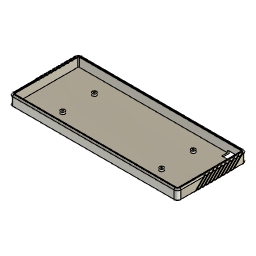
SpeedTray (Autodesk Fusion 360 design; units mm, degrees)
Autodesk Fusion 360 part; units mm, degrees
note: some values were not read from the file. Set by a fixed rule: which sketch regions a step uses.
sketch "Outline Sketch" plane through (0, 0, 0) normal (0, 0, 1) x (1, 0, 0)
  line L0 (16.7505, 7.3816) -> (212.013, 7.3816) construction
  line L1 (212.013, 7.3816) -> (212.013, 83.5816) construction
  line L2 (212.013, 83.5816) -> (16.7505, 83.5816) construction
  line L3 (16.7505, 83.5816) -> (16.7505, 7.3816) construction
  line L4 (212.513, 84.0816) -> (16.2505, 84.0816)
  line L5 (16.2505, 84.0816) -> (16.2505, 6.8816)
  line L6 (16.2505, 6.8816) -> (212.513, 6.8816)
  line L7 (212.513, 6.8816) -> (212.513, 84.0816)
  line L8 (13.0505, 3.6816) -> (215.713, 3.6816)
  line L9 (215.713, 3.6816) -> (215.713, 87.2816)
  line L10 (215.713, 87.2816) -> (13.0505, 87.2816)
  line L11 (13.0505, 87.2816) -> (13.0505, 3.6816)
  dimension "d1" = 195.2625
  dimension "d2" = 76.2
  dimension "d3" = 0.5
  dimension "d4" = 3.7
  constraint horizontal L0
  constraint vertical L1
  constraint horizontal L2
  constraint vertical L3
  measures "d1" distance of L0.start L0.end
  measures "d2" distance of L0.start L2.end
extrude "Extrude1" add sketch "Outline Sketch" along normal blind 8.6
sketch "Angle Sketch" plane through (215.713, 0, 0) normal (1, 0, 0) x (0, 1, 0)
  line L0 (3.6816, 0) -> (87.2816, 0)
  line L1 (87.2816, 0) -> (87.2816, 8.6)
  line L2 (87.2816, 8.6) -> (3.6816, 8.6)
  line L3 (3.6816, 8.6) -> (3.6816, 0)
  line L4 (3.6816, -4.2) -> (87.2816, -4.2)
  dimension "d20" = 4.2
ref_plane "WorkPlane1" through (215.713, 45.4816, -4.2) normal (0, 0, -1) x (0, 1, 0)
sketch "Sketch for Base" plane through (0, 0, 0) normal (0, 0, -1) x (1, 0, 0)
  line L0 (212.513, -6.8816) -> (212.513, -84.0816)
  line L1 (212.513, -84.0816) -> (16.2505, -84.0816)
  line L2 (16.2505, -84.0816) -> (16.2505, -6.8816)
  line L3 (16.2505, -6.8816) -> (212.513, -6.8816)
  line L4 (13.0505, -3.6816) -> (13.0505, -87.2816)
  line L5 (13.0505, -87.2816) -> (215.713, -87.2816)
  line L6 (215.713, -87.2816) -> (215.713, -3.6816)
  line L7 (215.713, -3.6816) -> (13.0505, -3.6816)
  line L8 (13.0505, -87.2816) -> (215.713, -87.2816)
  line L9 (215.713, -87.2816) -> (215.713, -3.6816)
  line L10 (215.713, -3.6816) -> (13.0505, -3.6816)
  line L11 (13.0505, -3.6816) -> (13.0505, -87.2816)
  constraint horizontal L8
  constraint vertical L9
  constraint horizontal L10
  constraint vertical L11
  constraint coincident L6.end L7.start
  constraint coincident L4.end L5.start
extrude "Extrude2" add sketch "Sketch for Base" along normal up to surface (4.2 mm away) contours L0 L1 L2 L3 | L4 L5 L6 L7 L8 L9 L10 L11
sketch "Hole and USB C Cutout Sketch" plane through (0, 0, 0) normal (0, 0, 1) x (-1, 0, 0)
  line L0 (-212.513, -84.0816) -> (-16.2505, -84.0816)
  line L1 (-16.2505, -84.0816) -> (-16.2505, -6.8816)
  line L2 (-16.2505, -6.8816) -> (-212.513, -6.8816)
  line L3 (-212.513, -6.8816) -> (-212.513, -84.0816)
  line L4 (-16.2505, -84.0816) -> (-54.8505, -84.0816) construction
  line L5 (-54.8505, -84.0816) -> (-54.8505, -64.5316) construction
  circle A0 centre (-54.8505, -64.5316) radius 2.5
  line L6 (-212.513, -84.0816) -> (-200.1067, -84.0816)
  line L7 (-195.3817, -87.2816) -> (-204.8317, -87.2816)
  line L8 (-204.8317, -87.2816) -> (-204.8317, -77.4816)
  line L9 (-204.8317, -77.4816) -> (-195.3817, -77.4816)
  line L10 (-195.3817, -77.4816) -> (-195.3817, -87.2816)
  line L11 (-200.1067, -84.0816) -> (-200.1067, -83.5816)
  circle A1 centre (-173.913, -64.5316) radius 2.5
  line L12 (-212.513, -6.8816) -> (-212.513, -84.0816)
  line L13 (-212.513, -84.0816) -> (-16.2505, -84.0816)
  circle A2 centre (-173.913, -26.4316) radius 2.5
  circle A3 centre (-54.8505, -26.4316) radius 2.5
  line L14 (-16.2505, -84.0816) -> (-16.2505, -6.8816)
  line L15 (-16.7505, -7.3816) -> (-212.013, -7.3816)
  line L16 (-16.2505, -6.8816) -> (-212.513, -6.8816)
  dimension "d17" = 38.6
  dimension "d18" = 19.55
  dimension "d19" = 5
  dimension "d21" = 12.4063
  dimension "d22" = 9.45
  dimension "d23" = 4.725
  dimension "d24" = 0.5
  dimension "d25" = 3.7
  dimension "d26" = 9.8
  dimension "d38" = 5
  dimension "d39" = 38.6
  dimension "d40" = 19.55
  dimension "d41" = 5
  dimension "d42" = 5
  dimension "d43" = 38.6
  dimension "d45" = 38.6
  dimension "d46" = 19.55
  dimension "d47" = 19.55
  constraint coincident L0.end L1.start
  constraint perpendicular L1 L4
  constraint perpendicular L4 L5
  constraint coincident L5.end A0.centre
  constraint coincident L0.start L3.end
  constraint perpendicular L3 L6
  constraint horizontal L7
  constraint vertical L8
  constraint horizontal L9
  constraint vertical L10
  constraint perpendicular L6 L11
  measures "d17" distance of L0.end L4.end
  measures "d18" distance of L4.end L5.end
  measures "d19" diameter of A0
  measures "d21" distance of L0.start L6.end
  measures "d22" distance of L8 L10
  measures "d23" distance of L6.end L8
  measures "d24" distance of L6.end L11.end
  measures "d25" distance of L7 L11.end
  measures "d26" distance of L7 L9
  measures "d38" diameter of A1
  measures "d39" distance of A1.centre L12
  measures "d40" distance of A1.centre L13
  measures "d41" diameter of A2
  measures "d42" diameter of A3
  measures "d43" distance of A3.centre L14
  measures "d45" distance of L12 A2.centre
  measures "d46" distance of A2.centre L16
  measures "d47" distance of A3.centre L16
extrude "Extrude3" cut sketch "Hole and USB C Cutout Sketch" along normal blind -6 and the other way blind -0.5 contours L0 L6 L8 L9 L10 L13 | L0 L6 L7 L8 L10 L13
extrude "Extrude4" cut sketch "Hole and USB C Cutout Sketch" against normal blind 2.4 contours L0 L1 L2 L3 L6 L8 L9 L10 L12 L13 L14 L16
fillet "Fillet6" radius 1 4 edges at (16.2505, 6.8816, 3.1) (16.2505, 84.0816, 3.1) (212.513, 84.0816, 3.1) (212.513, 6.8816, 3.1)
hole "Hole1" at (54.8505, 64.5316, 0) direction (0, 0, -1) diameter 1.8 depth 3 tip angle 180
hole "Hole2" at (54.8505, 26.4316, 0) direction (0, 0, -1) diameter 1.8 depth 3 tip angle 180
hole "Hole3" at (173.913, 64.5316, 0) direction (0, 0, -1) diameter 1.8 depth 3 tip angle 180
hole "Hole4" at (173.913, 26.4316, 0) direction (0, 0, -1) diameter 1.8 depth 3 tip angle 180
fillet "Fillet8" radius 4.2 4 edges at (13.0505, 3.6816, 2.2) (13.0505, 87.2816, 2.2) (215.713, 87.2816, 2.2) (215.713, 3.6816, 2.2)
sketch "Decoration Lines" plane through (215.713, 0, 0) normal (1, 0, 0) x (0, 1, 0)
  line L0 (7.8816, 8.6) -> (7.8816, -4.2)
  line L1 (7.8816, -4.2) -> (83.0816, -4.2)
  line L2 (83.0816, -4.2) -> (83.0816, 8.6)
  line L3 (83.0816, 8.6) -> (7.8816, 8.6)
  line L4 (83.0816, 8.6) -> (70.2816, -4.2)
  line L5 (83.0816, 8.6) -> (101.1835, 8.6) construction
  line L6 (83.0816, 8.6) -> (82.3745, 9.3071)
  line L7 (82.3745, 9.3071) -> (68.8674, -4.2)
  line L8 (82.3745, 9.3071) -> (101.4764, 9.3071) construction
  line L9 (68.8674, -4.2) -> (70.2816, -4.2)
  line L10 (78.0816, 8.6) -> (77.3745, 9.3071)
  line L11 (78.0816, 8.6) -> (65.2816, -4.2)
  line L12 (63.8674, -4.2) -> (65.2816, -4.2)
  line L13 (77.3745, 9.3071) -> (63.8674, -4.2)
  line L14 (73.0816, 8.6) -> (72.3745, 9.3071)
  line L15 (73.0816, 8.6) -> (60.2816, -4.2)
  line L16 (58.8674, -4.2) -> (60.2816, -4.2)
  line L17 (72.3745, 9.3071) -> (58.8674, -4.2)
  line L18 (68.0816, 8.6) -> (67.3745, 9.3071)
  line L19 (68.0816, 8.6) -> (55.2816, -4.2)
  line L20 (53.8674, -4.2) -> (55.2816, -4.2)
  line L21 (67.3745, 9.3071) -> (53.8674, -4.2)
  line L22 (63.0816, 8.6) -> (62.3745, 9.3071)
  line L23 (63.0816, 8.6) -> (50.2816, -4.2)
  line L24 (48.8674, -4.2) -> (50.2816, -4.2)
  line L25 (62.3745, 9.3071) -> (48.8674, -4.2)
  line L26 (58.0816, 8.6) -> (57.3745, 9.3071)
  line L27 (58.0816, 8.6) -> (45.2816, -4.2)
  line L28 (43.8674, -4.2) -> (45.2816, -4.2)
  line L29 (57.3745, 9.3071) -> (43.8674, -4.2)
  line L30 (53.0816, 8.6) -> (52.3745, 9.3071)
  line L31 (53.0816, 8.6) -> (40.2816, -4.2)
  line L32 (38.8674, -4.2) -> (40.2816, -4.2)
  line L33 (52.3745, 9.3071) -> (38.8674, -4.2)
  line L34 (48.0816, 8.6) -> (47.3745, 9.3071)
  line L35 (48.0816, 8.6) -> (35.2816, -4.2)
  line L36 (33.8674, -4.2) -> (35.2816, -4.2)
  line L37 (47.3745, 9.3071) -> (33.8674, -4.2)
  line L38 (43.0816, 8.6) -> (42.3745, 9.3071)
  line L39 (43.0816, 8.6) -> (30.2816, -4.2)
  line L40 (28.8674, -4.2) -> (30.2816, -4.2)
  line L41 (42.3745, 9.3071) -> (28.8674, -4.2)
  line L42 (38.0816, 8.6) -> (37.3745, 9.3071)
  line L43 (38.0816, 8.6) -> (25.2816, -4.2)
  line L44 (23.8674, -4.2) -> (25.2816, -4.2)
  line L45 (37.3745, 9.3071) -> (23.8674, -4.2)
  line L46 (83.0816, 8.6) -> (81.6674, 8.6)
  line L47 (82.0816, 7.6) -> (35.6674, 7.6)
  dimension "d139" = 135
  dimension "d140" = 1
  dimension "d141" = 135
  dimension "d144" = -5
  dimension "d145" = 0
  dimension "d170" = 1
  constraint horizontal L5
  constraint coincident L2.end L3.start
  constraint coincident L1 L4.end
  constraint perpendicular L4 L6
  constraint horizontal L8
  constraint coincident L1 L7.end
  constraint coincident L7 L46.end
  constraint coincident L3 L46.end
  constraint perpendicular L2 L47
  constraint coincident L45 L47.end
  constraint coincident L4 L47.start
  measures "d139" angle of L4 L5
  measures "d140" distance of L2.end L6.end
  measures "d141" angle of L7 L8
  measures "d170" distance of L46 L47
fillet "Fillet10" radius 1.5 8 edges at (214.4828, 86.0514, 8.6) (215.713, 45.4816, 8.6) (214.4828, 4.9117, 8.6) (114.3817, 3.6816, 8.6) (14.2806, 4.9117, 8.6) (13.0505, 45.4816, 8.6) (14.2806, 86.0514, 8.6) (114.3817, 87.2816, 8.6)
fillet "Fillet15" radius 1.5 9 edges at (106.3161, 87.2816, -4.2) (14.2806, 86.0514, -4.2) (13.0505, 45.4816, -4.2) (14.2806, 4.9117, -4.2) (114.3817, 3.6816, -4.2) (214.4828, 4.9117, -4.2) (215.713, 45.4816, -4.2) (214.4828, 86.0514, -4.2) (208.1723, 87.2816, -4.2)
chamfer "Chamfer5" distance 0.5 angle 45 8 edges at (114.3817, 84.0816, 8.6) (212.2201, 83.7887, 8.6) (212.513, 45.4816, 8.6) (212.2201, 7.1745, 8.6) (114.3817, 6.8816, 8.6) (16.5434, 7.1745, 8.6) (16.2505, 45.4816, 8.6) (16.5434, 83.7887, 8.6)
extrude "Extrude13" cut sketch "Decoration Lines" against normal blind 1 contours L3 L43 L45 L47 | L1 L43 L44 L45 L47 | L3 L39 L41 L47 | L1 L39 L40 L41 L47 | L3 L35 L37 L47 | L1 L35 L36 L37 L47 | L3 L31 L33 L47 | L1 L31 L32 L33 L47 | L3 L27 L29 L47 | L1 L27 L28 L29 L47 | L3 L23 L25 L47 | L1 L23 L24 L25 L47 | L3 L19 L21 L47 | L1 L19 L20 L21 L47 | L3 L15 L17 L47 | L1 L15 L16 L17 L47 | L3 L11 L13 L47 | L1 L11 L12 L13 L47 | L3 L4 L7 L46 L47 | L1 L4 L7 L9 L47
extrude "Extrude17" cut sketch "Decoration Lines" against normal blind 5 contours L3 L43 L45 L47 | L3 L39 L41 L47 | L3 L35 L37 L47 | L3 L31 L33 L47 | L3 L27 L29 L47 | L3 L23 L25 L47 | L3 L19 L21 L47 | L3 L15 L17 L47 | L3 L11 L13 L47 | L3 L4 L7 L46 L47
extrude "Extrude14" cut sketch "Decoration Lines" along normal blind 1 from surface at -202.6625 contours L3 L43 L45 L47 | L1 L43 L44 L45 L47 | L3 L39 L41 L47 | L1 L39 L40 L41 L47 | L3 L35 L37 L47 | L1 L35 L36 L37 L47 | L3 L31 L33 L47 | L1 L31 L32 L33 L47 | L3 L27 L29 L47 | L1 L27 L28 L29 L47 | L3 L23 L25 L47 | L1 L23 L24 L25 L47 | L3 L19 L21 L47 | L1 L19 L20 L21 L47 | L3 L15 L17 L47 | L1 L15 L16 L17 L47 | L3 L11 L13 L47 | L1 L11 L12 L13 L47 | L3 L4 L7 L46 L47 | L1 L4 L7 L9 L47
extrude "Extrude18" cut sketch "Decoration Lines" along normal blind 5 from surface at -202.6625 contours L3 L43 L45 L47 | L3 L39 L41 L47 | L3 L35 L37 L47 | L3 L31 L33 L47 | L3 L27 L29 L47 | L3 L23 L25 L47 | L3 L19 L21 L47 | L3 L15 L17 L47 | L3 L11 L13 L47 | L3 L4 L7 L46 L47
sketch "Sketch10" plane through (0, 87.2816, 0) normal (0, 1, 0) x (-1, 0, 0)
  line L0 (-211.513, 7.1) -> (-211.513, -2.7)
  line L1 (-204.8317, -2.7) -> (-204.8317, 0.5)
  line L2 (-204.8317, 0.5) -> (-195.3817, 0.5)
  line L3 (-195.3817, 0.5) -> (-195.3817, -2.7)
  line L4 (-17.2505, -2.7) -> (-17.2505, 7.1)
  line L5 (-17.2505, 7.1) -> (-211.513, 7.1)
  line L6 (-211.513, -2.7) -> (-204.8317, -2.7)
  line L7 (-195.3817, -2.7) -> (-17.2505, -2.7)
  line L8 (-204.8317, 0.25) -> (-195.3817, 0.25) construction
  line L9 (-195.3817, 0.25) -> (-195.3817, -3.41) construction
  line L10 (-195.3817, -3.41) -> (-204.8317, -3.41) construction
  line L11 (-204.8317, -3.41) -> (-204.8317, 0.25) construction
  line L12 (-204.8317, -3.41) -> (-195.3817, 0.25) construction
  line L13 (-204.8317, 0.25) -> (-195.3817, -3.41) construction
  line L14 (-196.9317, 2.5) -> (-203.2817, 2.5)
  line L15 (-207.0817, -1.3) -> (-207.0817, -1.86)
  line L16 (-203.2817, -5.66) -> (-196.9317, -5.66)
  line L17 (-193.1317, -1.86) -> (-193.1317, -1.3)
  line L18 (-193.1317, 2.5) -> (-207.0817, -5.66) construction
  line L19 (-207.0817, 2.5) -> (-193.1317, -5.66) construction
  arc A0 (-203.2817, 2.5) -> (-207.0817, -1.3) centre (-203.2817, -1.3) ccw
  arc A1 (-193.1317, -1.3) -> (-196.9317, 2.5) centre (-196.9317, -1.3) ccw
  arc A2 (-196.9317, -5.66) -> (-193.1317, -1.86) centre (-196.9317, -1.86) ccw
  arc A3 (-207.0817, -1.86) -> (-203.2817, -5.66) centre (-203.2817, -1.86) ccw
  point P0 (-200.1067, -1.58)
  dimension "d180" = 9.45
  dimension "d181" = 3.66
  dimension "d182" = 0.25
  dimension "d183" = 13.95
  dimension "d184" = 8.16
  dimension "d185" = 3.8
  constraint horizontal L8
  constraint vertical L9
  constraint horizontal L10
  constraint vertical L11
  constraint collinear L3 L9
  constraint horizontal L14
  constraint perpendicular L14 L15
  constraint parallel L14 L16
  constraint parallel L15 L17
  constraint coincident L18 P0
  constraint coincident L19 P0
  constraint midpoint L12 P0
  constraint coincident L19.start L15
  constraint coincident L19.start L14
  constraint tangent L15 A0
  constraint tangent L14 A0
  constraint coincident L18.start L14
  constraint coincident L18.start L17
  constraint tangent L14 A1
  constraint tangent L17 A1
  constraint equal A0 A1
  constraint coincident L19.end L17
  constraint coincident L19.end L16
  constraint tangent L17 A2
  constraint tangent L16 A2
  constraint equal A0 A2
  constraint coincident L18.end L16
  constraint coincident L18.end L15
  constraint tangent L16 A3
  constraint tangent L15 A3
  constraint equal A0 A3
  measures "d180" distance of L8.start L8.end
  measures "d181" distance of L8.start L10.end
  measures "d182" distance of L2 L8
  measures "d183" distance of L18.end L19.end
  measures "d184" distance of L19.start L18.end
  measures "d185" radius of A0
extrude "Extrude16" cut sketch "Sketch10" against normal blind 1 contours L1 L2 L3 L6 L7 L14 L15 L17 A0 A1 A2 A3 | L1 L2 L3 L6 L7 L16 A2 A3
fillet "Fillet19" radius 1.55 2 edges at (204.8317, 85.1816, 0.5) (195.3817, 85.1816, 0.5)
fillet "Fillet18" radius 1.5 10 edges at (214.713, 36.3745, 7.6) (214.713, 41.3745, 7.6) (214.713, 46.3745, 7.6) (214.713, 51.3745, 7.6) (214.713, 56.3745, 7.6) (214.713, 61.3745, 7.6) (214.713, 66.3745, 7.6) (214.713, 71.3745, 7.6) (214.713, 76.3745, 7.6) (214.713, 81.3745, 7.6)
fillet "Fillet18" radius 1.5 10 edges at (14.0505, 36.3745, 7.6) (14.0505, 41.3745, 7.6) (14.0505, 46.3745, 7.6) (14.0505, 51.3745, 7.6) (14.0505, 56.3745, 7.6) (14.0505, 61.3745, 7.6) (14.0505, 66.3745, 7.6) (14.0505, 71.3745, 7.6) (14.0505, 81.3745, 7.6) (14.0505, 76.3745, 7.6)
equation "d1 = 19.05 mm * 10.25"
equation "d2 = 19.05 mm * 4"
equation "d5 = 7.6 mm + 1 mm"
equation "d17 = 19.05 mm * 2 + 0.5 mm"
equation "d18 = 19.05 mm + 0.5 mm"
equation "d21 = 19.05 mm * 0.625 + 0.5 mm"
equation "d23 = d22 / 2"
equation "d25 = d4"
equation "d26 = 1.9 mm + 7.9 mm"
equation "d39 = d17"
equation "d40 = d18"
equation "d43 = d17"
equation "d45 = d17"
equation "d46 = d18"
equation "d47 = d18"
equation "d64 = d4 - 0.5 mm"
named bodies: "KS-33 QAZ"
